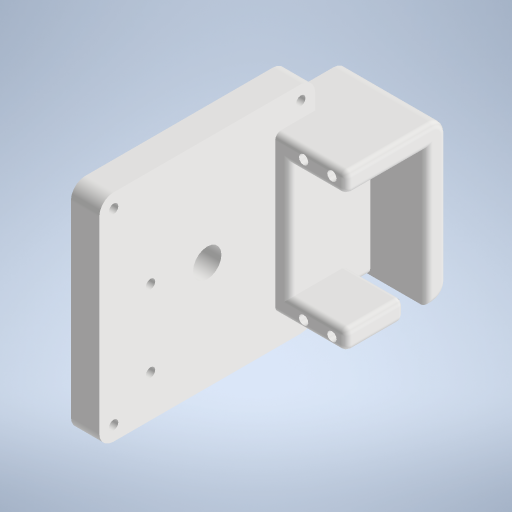
# Autodesk Inventor part: separator_plate
Saved by Autodesk Inventor 2023 (Build 270158000, 158)
## iProperties
Created: 2023-01-24
Part Number: separator_plate
Material: Generic
Document SubType Name: Modeling
Designer: Hunter
Density: 1 g/cm^3
Appearance: Default
Author: Hunter
Autodesk Inventor part; units mm, degrees
ref_plane "YZ Plane" through (0, 0, 0) normal (1, 0, 0) x (0, 1, 0)
ref_plane "XZ Plane" through (0, 0, 0) normal (0, 1, 0) x (-1, 0, 0)
ref_plane "XY Plane" through (0, 0, 0) normal (0, 0, 1) x (1, 0, 0)
sketch "Sketch1" plane through (0, 0, 0) normal (1, 0, 0) x (0, 1, 0)
  line L0 (0, 42.25) -> (-55, 42.25)
  line L1 (-55, 42.25) -> (-55, -42.25)
  line L2 (-55, -42.25) -> (0, -42.25)
  line L3 (0, -42.25) -> (0, 42.25)
  point P0 (0, 0)
  point P1 (0, 0)
  dimension "d0" = 84.5
  dimension "d1" = 55
  constraints: 8 end point, 2 parallel, 1 coincident, 1 horizontal, 1 midpoint, 1 perpendicular
  measures "d0" distance of L2.end L0.start
  measures "d1" distance of L0.start L0.end
extrude "Extrusion1" add sketch "Sketch1" along normal blind 10
sketch "Sketch2" plane through (10, 0, 0) normal (1, 0, 0) x (0, 0, -1)
  line L0 (42.25, -55) -> (42.25, 0) projected
  line L1 (-42.25, -55) -> (42.25, -55) projected
  line L2 (42.25, 0) -> (35.25, 0)
  line L3 (35.25, 0) -> (35.25, -55)
  line L4 (35.25, -55) -> (42.25, -55)
  line L5 (42.25, -55) -> (42.25, 0)
  line L6 (35.25, 0) -> (6.75, 0)
  line L7 (6.75, 0) -> (6.75, -7)
  line L8 (6.75, -7) -> (35.25, -7)
  line L9 (35.25, -7) -> (35.25, 0)
  line L10 (35.25, -55) -> (6.75, -55)
  line L11 (6.75, -55) -> (6.75, -48)
  line L12 (6.75, -48) -> (35.25, -48)
  line L13 (35.25, -48) -> (35.25, -55)
  line L14 (6.75, -7) -> (35.25, -7)
  line L15 (35.25, -7) -> (35.25, -48)
  line L16 (35.25, -48) -> (6.75, -48)
  line L17 (6.75, -48) -> (6.75, -7)
  point P0 (0, 0)
  point P1 (35.25, -7)
  point P2 (35.25, -48)
  point P3 (6.75, -55)
  dimension "d11" = 7
  dimension "d12" = 28.5
  dimension "d13" = 7
  dimension "d14" = 28.5
  dimension "d15" = 7
  constraints: 32 end point, 8 parallel, 4 horizontal, 4 perpendicular, 1 point on line
  measures "d11" distance of L0.end L2.end
  measures "d12" distance of L7.end L8.end
  measures "d13" distance of L6.end L7.end
  measures "d14" distance of L11.end L12.end
  measures "d15" distance of L10.end L11.end
extrude "Extrusion2" add sketch "Sketch2" along normal blind 25 contours L1 L3 L2 L0 | L1 L11 L12 L3 | L3 L8 L7 L6
extrude "Extrusion3" add sketch "Sketch2" along normal blind 5 contours L12 L17 L8 L3
sketch "Sketch4" plane through (0, -55, -42.25) normal (0, -1, 0) x (1, 0, 0)
  line L0 (15, 7) -> (15, 35.5) projected
  line L1 (35, 7) -> (35, 35.5) projected
  line L2 (15, 7) -> (35, 7) projected
  line L3 (15, 7) -> (35, 7) projected
  line L4 (35, 7) -> (15, 7)
  line L5 (15, 7) -> (15, 15)
  line L6 (15, 15) -> (35, 15)
  line L7 (35, 15) -> (35, 7)
  point P0 (0, 42.25)
  dimension "d27" = 8
  constraints: 8 end point, 2 parallel, 1 horizontal, 1 perpendicular, 1 point on line
  measures "d27" distance between parallel lines of L2 L6
extrude "Extrusion5" cut sketch "Sketch4" against normal up to surface (7 mm away)
sketch "Sketch5" plane through (10, -55, -6.75) normal (0, 0, 1) x (1, 0, 0)
  circle A0 centre (10, 52) radius 1.65
  circle A1 centre (20, 52) radius 1.65
  circle A2 centre (10, 3) radius 1.65
  circle A3 centre (20, 3) radius 1.65
  line L0 (5, 48) -> (5, 7) projected
  line L1 (5, 48) -> (25, 48) projected
  line L2 (5, 7) -> (25, 7) projected
  point P0 (-10, 55)
  dimension "d29" = 5
  dimension "d30" = 4
  dimension "d31" = 3.3
  dimension "d32" = 4
  dimension "d34" = 10
  constraints: 4 centre point, 3 equal radius, 2 horizontal alignment, 2 vertical alignment
  measures "d29" distance from line of L0 A0.centre
  measures "d30" distance from line of L1 A0.centre
  measures "d31" diameter of A0
  measures "d32" distance from line of L2 A2.centre
  measures "d34" distance of A1.centre A0.centre
extrude "Extrusion6" cut sketch "Sketch5" against normal up to surface (28.5 mm away)
fillet "Fillet2" radius 5 4 edges at (5, -55, 42.25) (5, 0, 42.25) (17.5, -55, -42.25) (17.5, 0, -42.25)
sketch "Sketch8" plane through (0, 0, 0) normal (-1, 0, 0) x (0, 0, 1)
  line L0 (37.25, -55) -> (-37.25, -55) construction
  line L1 (0, -55) -> (0, 0) construction
  line L2 (42.25, -5) -> (42.25, -50) construction
  line L3 (-42.25, -50) -> (-42.25, -5) construction
  circle A0 centre (17.25, -27.5) radius 10.5
  circle A1 centre (17.25, -27.5) radius 5
  line L4 (-37.25, 0) -> (37.25, 0) projected
  circle A2 centre (17.25, -27.5) radius 11.5
  dimension "d55" = 21
  dimension "d56" = 10
  dimension "d70" = 25
  dimension "d71" = 27.5
  dimension "d86" = 23
  constraints: 3 centre point, 2 coincident, 2 end point, 1 midpoint, 1 vertical
  measures "d55" diameter of A0
  measures "d56" diameter of A1
  measures "d70" distance from line of L2 A0.centre
  measures "d71" distance from line of L4 A0.centre
  measures "d86" diameter of A2
extrude "Extrusion8" add sketch "Sketch8" along normal blind 2 contours A2
extrude "Extrusion9" cut sketch "Sketch8" against normal through all contours A1
fillet "Fillet3" radius 2 16 edges at (35, -51.5, -6.75) (35, -51.5, -27.25) (35, -3.5, -6.75) (25, -7, -6.75) (22.5, 0, -6.75) (25, -48, -6.75) (22.5, -55, -6.75) (25, -55, -27.25) (25, -48, -27.25) (35, -31, -35.25) (35, -7, -21) (35, -1.4645, -40.7855) (35, 0, -22) (35, -53.5355, -40.7855) (35, -55, -36.25) (35, -27.5, -42.25)
fillet "Fillet4" radius 2 6 edges at (34.4142, -54.4142, -26.6642) (34.4142, -54.4142, -7.3358) (35, -55, -17) (34.4142, -48.5858, -7.3358) (34.4142, -48.5858, -26.6642) (35, -48, -17)
fillet "Fillet5" radius 2 2 edges at (15, -27.5, -6.75) (15, -55, -30.25)
sketch "Sketch9" plane through (10, 0, 0) normal (1, 0, 0) x (0, 0, -1)
  circle A0 centre (-37.25, -24) radius 1.65
  circle A1 centre (-37.25, -51) radius 1.65
  line L0 (-37.25, -55) -> (8.75, -55) projected
  line L1 (-42.25, -5) -> (-42.25, -50) projected
  point P0 (0, 0)
  dimension "d64" = 27
  dimension "d65" = 3.3
  dimension "d66" = 4
  dimension "d67" = 5
  constraints: 2 centre point, 1 equal radius, 1 vertical alignment
  measures "d64" distance of A1.centre A0.centre
  measures "d65" diameter of A0
  measures "d66" distance from line of L0 A1.centre
  measures "d67" distance from line of L1 A1.centre
extrude "Extrusion10" cut sketch "Sketch9" against normal through all
sketch "Sketch10" plane through (10, 0, 0) normal (1, 0, 0) x (0, 0, -1)
  circle A0 centre (-17.25, -27.5) radius 5 construction
  line L0 (-55.35, -65.6) -> (20.85, -65.6)
  line L1 (20.85, -65.6) -> (20.85, 10.6)
  line L2 (20.85, 10.6) -> (-55.35, 10.6)
  line L3 (-55.35, 10.6) -> (-55.35, -65.6)
  line L4 (-55.35, -65.6) -> (20.85, 10.6) construction
  line L5 (20.85, -65.6) -> (-55.35, 10.6) construction
  circle A1 centre (15.77, -60.52) radius 1.65
  circle A2 centre (-50.27, -60.52) radius 1.65
  circle A3 centre (-50.27, 5.52) radius 1.65
  circle A4 centre (15.77, 5.52) radius 1.65
  line L6 (-37.25, -55) -> (8.75, -55) projected
  arc A5 (-42.25, -50) -> (-37.25, -55) centre (-37.25, -50) ccw projected
  line L7 (-42.25, -5) -> (-42.25, -50) projected
  arc A6 (-37.25, 0) -> (-42.25, -5) centre (-37.25, -5) ccw projected
  line L8 (8.75, 0) -> (-37.25, 0) projected
  line L9 (8.75, -55) -> (25.25, -55) projected
  line L10 (37.25, 0) -> (8.75, 0) projected
  point P0 (0, 0)
  point P1 (20.85, -55)
  point P2 (20.85, 0)
  dimension "d72" = 76.2
  dimension "d73" = 76.2
  dimension "d74" = 3.3
  dimension "d75" = 5.08
  constraints: 12 end point, 4 centre point, 4 point on line, 3 equal radius, 2 horizontal alignment, 2 midpoint, 2 parallel, 2 vertical alignment, 1 horizontal, 1 perpendicular
  measures "d72" distance of L2.end L1.end
  measures "d73" distance of L2.end L0.start
  measures "d74" diameter of A2
  measures "d75" distance from line of L3 A2.centre
extrude "Extrusion11" add sketch "Sketch10" against normal blind 10 contours L3 L2 L1 L10 L8 A6 L7 A5 L6 L9 L0
fillet "Fillet6" radius 5 4 edges at (5, -65.6, 55.35) (5, -65.6, -20.85) (5, 10.6, 55.35) (5, 10.6, -20.85)
body "Solid1"
